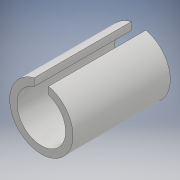
# Autodesk Inventor part: leverHook
Saved by Autodesk Inventor 2018 (Build 220112000, 112)
## iProperties
Created: 2018-11-25
Part Number: leverHook
Material: Generic
Document SubType Name: Modeling
Designer: Prakash
Density: 1 g/cm^3
Appearance: Default
Author: Prakash
Autodesk Inventor part; units mm, degrees
ref_plane "YZ Plane" through (0, 0, 0) normal (1, 0, 0) x (0, 1, 0)
ref_plane "XZ Plane" through (0, 0, 0) normal (0, 1, 0) x (-1, 0, 0)
ref_plane "XY Plane" through (0, 0, 0) normal (0, 0, 1) x (1, 0, 0)
sketch "Sketch1" plane through (0, 0, 0) normal (0, 1, 0) x (-1, 0, 0)
  arc A0 (-1.5, 4.7697) -> (1.5, 4.7697) centre (0, 0) ccw
  arc A1 (-1.5, 6.3246) -> (1.5, 6.3246) centre (0, 0) ccw
  line L0 (0, 5) -> (0, 0) construction
  line L1 (1.5, 4.7697) -> (1.5, 6.3246)
  line L2 (-1.5, 4.7697) -> (-1.5, 6.3246)
  dimension "d0" = 10
  dimension "d1" = 13
  dimension "d5" = 3
  constraints: 6 end point, 4 point on circle, 2 centre point, 2 coincident, 2 vertical, 1 parallel, 1 other
  measures "d0" diameter of A0
  measures "d1" diameter of A1
  measures "d5" distance between parallel lines of L2 L1
extrude "Extrusion1" add sketch "Sketch1" along normal blind 20
body "Solid1"
